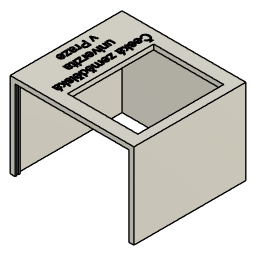
vrchni kryt (Autodesk Fusion 360 design; units mm, degrees)
Autodesk Fusion 360 part; units mm, degrees
note: some values were not read from the file. Set by a fixed rule: which sketch regions a step uses.
sketch "Sketch1" plane through (0, 0, 0) normal (0, 0, 1) x (1, 0, 0)
  line L0 (0, 0) -> (113.6, 0)
  line L1 (113.6, 0) -> (113.6, 101.8)
  line L2 (113.6, 101.8) -> (0, 101.8)
  line L3 (0, 101.8) -> (0, 0)
  line L4 (115.6, 0) -> (115.6, 103.8)
  line L5 (115.6, 103.8) -> (-2, 103.8)
  line L6 (-2, 103.8) -> (-2, 0)
  line L7 (118.6, 0) -> (118.6, 106.8)
  line L8 (118.6, 106.8) -> (-5, 106.8)
  line L9 (-5, 106.8) -> (-5, 0)
  line L10 (39.5, 93.8) -> (109.5, 93.8)
  line L11 (109.5, 93.8) -> (109.5, 8)
  line L12 (109.5, 8) -> (39.5, 8)
  line L13 (39.5, 8) -> (39.5, 93.8)
  line L14 (10, 90) -> (10, 10) construction
  line L15 (10, 10) -> (50, 10) construction
  line L16 (50, 10) -> (50, 90) construction
  line L17 (50, 90) -> (10, 90) construction
  line L18 (0, 0) -> (-5, 0)
  line L19 (113.6, 0) -> (118.6, 0)
  line L20 (118.6, 0) -> (113.6, 0)
  line L21 (113.6, -5) -> (118.6, -5)
  line L22 (118.6, -5) -> (118.6, 0)
  line L23 (-5, 0) -> (0, 0)
  line L24 (0, -5) -> (-5, -5)
  line L25 (-5, -5) -> (-5, 0)
  line L26 (0, -1.7) -> (-3.3, -1.7)
  line L27 (-3.3, -1.7) -> (-3.3, -3.3)
  line L28 (-3.3, -3.3) -> (0, -3.3)
  line L29 (0, 0) -> (0, -1.7)
  line L30 (0, -3.3) -> (0, -5)
  line L31 (116.9, -1.7) -> (113.6, -1.7)
  line L32 (113.6, -3.3) -> (116.9, -3.3)
  line L33 (116.9, -3.3) -> (116.9, -1.7)
  line L34 (113.6, 0) -> (113.6, -1.7)
  line L35 (113.6, -3.3) -> (113.6, -5)
  dimension "d3" = 113.6
  dimension "d4" = 101.8
  dimension "d9" = 9.1
  dimension "d10" = 70
  dimension "d12" = 13
  dimension "d13" = 7
  dimension "d19" = 5
  dimension "d20" = 5
  dimension "d21" = 5
  dimension "d22" = 5
  dimension "d23" = 1.6
  dimension "d24" = 1.7
  dimension "d25" = 1.7
  dimension "d26" = 1.6
  dimension "d27" = 1.7
  dimension "d28" = 1.7
  constraint horizontal L0
  constraint vertical L1
  constraint horizontal L2
  constraint vertical L3
  constraint coincident L0.start L3.end
  constraint horizontal L10
  constraint vertical L11
  constraint horizontal L12
  constraint vertical L13
  constraint perpendicular L9 L18
  constraint perpendicular L7 L19
  constraint coincident L18 L6.end
  constraint coincident L19 L4.start
  constraint horizontal L20
  constraint vertical L34
  constraint horizontal L21
  constraint vertical L22
  constraint horizontal L23
  constraint vertical L29
  constraint horizontal L24
  constraint vertical L25
  constraint horizontal L26
  constraint vertical L27
  constraint horizontal L28
  constraint collinear L29 L30
  constraint horizontal L31
  constraint horizontal L32
  constraint vertical L33
  constraint coincident L32.start L34
  constraint collinear L34 L35
  measures "d3" distance of L0.start L0.end
  measures "d4" distance of L0.end L1.end
  measures "d9" distance of L7 L11
  measures "d10" distance of L10.start L10.end
  measures "d12" distance of L8 L10
  measures "d19" distance of L7.start L0.end
  measures "d20" distance of L7.start L21.end
  measures "d21" distance of L9.end L0.start
  measures "d22" distance of L9.end L24.end
  measures "d23" distance of L26.start L28.end
  measures "d24" distance of L23 L26
  measures "d25" distance of L25 L27
  measures "d26" distance of L31.start L32.end
  measures "d27" distance of L19 L31
  measures "d28" distance of L22 L33
extrude "Extrude1" add sketch "Sketch1" along normal blind 5 contours L0 L1 L2 L3 | L1 L2 L3 L4 L5 L6 L18 L19 L20 L23 | L4 L5 L6 L7 L8 L9 L18 L19 L20 L23
extrude "Extrude2" add sketch "Sketch1" against normal blind 80 contours L18 L23 L24 L25 L26 L27 L28 L29 L30 | L19 L20 L21 L22 L31 L32 L33 L34 L35 | L4 L5 L6 L7 L8 L9 L18 L19 L20 L23
sketch "Sketch2" plane through (0, 0, 5) normal (0, 0, 1) x (-1, 0, 0)
  line L0 (-109.5, -8) -> (-39.5, -8)
  line L1 (-39.5, -8) -> (-39.5, -93.8)
  line L2 (-39.5, -93.8) -> (-109.5, -93.8)
  line L3 (-109.5, -93.8) -> (-109.5, -8)
  line L4 (5, -106.8) -> (5, 0)
  line L5 (-118.6, 0) -> (-118.6, -106.8)
  line L6 (-118.6, -106.8) -> (5, -106.8)
  line L7 (5, -100) -> (5, -5) construction
  line L8 (5, -5) -> (-40, -5) construction
  line L9 (-40, -5) -> (-40, -100) construction
  line L10 (-40, -100) -> (5, -100) construction
  line L11 (5, 0) -> (-118.6, 0)
  dimension "d14" = 8
  text T0 "Česká zemědělská univerzita\nv Praze" font "Arial" height 8 align centre middle in box 95 x 45 at (5, -100) x (0, 1) y (-1, 0) spacing 1
  constraint coincident L4
extrude "Extrude3" cut sketch "Sketch2" against normal blind 2 text T0
move_body "Move1" bodies 1 to x (1, 0, 0) y (0, 1, 0) z (0, 0, 1) at (0, 0, 80)
sketch "Sketch3" plane through (-5, 0, 0) normal (-1, 0, 0) x (0, -1, 0)
  line L0 (0, 80) -> (0, 85)
  line L1 (0, 85) -> (-106.8, 85)
  line L2 (-106.8, 85) -> (-106.8, 0)
  line L3 (-106.8, 0) -> (5, 0)
  line L4 (5, 0) -> (5, 80)
  line L5 (5, 80) -> (0, 80)
  line L6 (0, 80) -> (5, 80)
  line L7 (5, 80) -> (5, 85)
  line L8 (5, 85) -> (0, 85)
  line L9 (0, 85) -> (0, 80)
  line L10 (1.7, 80) -> (3.3, 80)
  line L11 (3.3, 80) -> (3.3, 83.3)
  line L12 (3.3, 83.3) -> (1.7, 83.3)
  line L13 (1.7, 83.3) -> (1.7, 80)
  dimension "d29" = 5
  dimension "d30" = 5
  dimension "d31" = 1.7
  dimension "d32" = 1.7
  dimension "d33" = 1.6
  constraint horizontal L6
  constraint vertical L7
  constraint horizontal L8
  constraint vertical L9
  constraint coincident L0.start L5.end
  constraint horizontal L10
  constraint vertical L11
  constraint horizontal L12
  constraint vertical L13
  constraint coincident L5 L10.start
  measures "d29" distance of L0.start L4.end
  measures "d30" distance of L0.start L0.end
  measures "d31" distance of L8 L12
  measures "d32" distance of L7 L11
  measures "d33" distance of L11 L13
extrude "Extrude5" add sketch "Sketch3" against normal blind 123.6 contours L0 L5 L6 L7 L8 L9 L11 L12 L13
sketch "Sketch4" plane through (-5, 0, 0) normal (-1, 0, 0) x (0, -1, 0)
  line L0 (5, 85) -> (-106.8, 85)
  line L1 (-106.8, 85) -> (-106.8, 0)
  line L2 (-106.8, 0) -> (5, 0)
  line L3 (5, 0) -> (5, 85)
  line L4 (1.7, 80) -> (1.7, 83.3)
  line L5 (1.7, 83.3) -> (3.3, 83.3)
  line L6 (3.3, 83.3) -> (3.3, 80)
  line L7 (3.3, 80) -> (1.7, 80)
extrude "Extrude6" add sketch "Sketch4" against normal blind 1.7 contours L4 L5 L6 L7
extrude "Extrude7" add 1 faces at (118.0333, -2.2333, 80) along direction (0, 0, 1) blind 3.3
